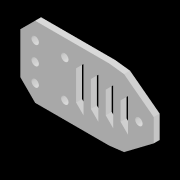
# Autodesk Inventor part: UpperArmMount
Saved by Autodesk Inventor 2020 (Build 240168000, 168)
## iProperties
Created: 2020-03-28
Part Number: UpperArmMount
Material: Generic
Document SubType Name: Modeling
Designer: valer
Density: 1 g/cm^3
Appearance: Default
Author: valer
Autodesk Inventor part; units mm, degrees
ref_plane "YZ Plane" through (0, 0, 0) normal (1, 0, 0) x (0, 1, 0)
ref_plane "XZ Plane" through (0, 0, 0) normal (0, 1, 0) x (-1, 0, 0)
ref_plane "XY Plane" through (0, 0, 0) normal (0, 0, 1) x (1, 0, 0)
sketch "Base" plane through (0, 0, 0) normal (0, 0, 1) x (1, 0, 0)
  line L0 (76.2, -12.7) -> (76.2, -19.05)
  line L1 (0, 0) -> (76.2, 0)
  line L2 (76.2, 0) -> (76.2, -60.96)
  line L3 (76.2, -60.96) -> (0, -60.96)
  line L4 (0, -60.96) -> (0, 0)
  line L5 (76.2, 0) -> (88.9, -1.5594)
  line L6 (88.9, -1.5594) -> (114.3, -20.6996)
  line L7 (114.3, -20.6996) -> (114.3, -30.48)
  line L8 (0, -30.48) -> (114.3, -30.48) construction
  line L9 (76.2, -60.96) -> (88.9, -59.4006)
  line L10 (88.9, -59.4006) -> (114.3, -40.2604)
  line L11 (114.3, -40.2604) -> (114.3, -30.48)
  circle A0 centre (12.7, -46.355) radius 3.175
  circle A1 centre (38.1, -46.355) radius 3.175
  circle A2 centre (38.1, -14.605) radius 3.175
  circle A3 centre (12.7, -14.605) radius 3.175
  line L12 (12.7, -46.355) -> (38.1, -46.355) construction
  line L13 (38.1, -46.355) -> (38.1, -14.605) construction
  line L14 (38.1, -14.605) -> (12.7, -14.605) construction
  line L15 (12.7, -14.605) -> (12.7, -46.355) construction
  circle A4 centre (12.7, -30.48) radius 3.175
  circle A5 centre (101.6, -30.48) radius 3.175
  point P0 (76.2, -30.48)
  dimension "d2" = 76.2
  dimension "d3" = 60.96
  dimension "d4" = 38.1
  dimension "d5" = 12.7
  dimension "d6" = 127
  dimension "d7" = 150
  dimension "d56" = 31.75
  dimension "d57" = 25.4
  dimension "d58" = 12.7
  dimension "d59" = 14.605
  dimension "d60" = 14.605
  dimension "d61" = 6.35
  dimension "d62" = 6.35
  dimension "d63" = 12.7
  constraints: 32 end point, 6 centre point, 4 parallel, 3 coincident, 3 midpoint, 3 point on line, 3 symmetric about line, 2 horizontal, 2 perpendicular, 1 vertical
  measures "d2" distance between parallel lines of L0 L4
  measures "d3" distance of L3.end L1.start
  measures "d4" distance from line of L2 L7.end
  measures "d5" horizontal distance of L1.end L5.end
  measures "d6" angle of L7 L6
  measures "d7" angle of L6 L5
  measures "d56" distance of L14.end L12.start
  measures "d57" distance of L12.start L12.end
  measures "d58" distance between parallel lines of L4 L15
  measures "d59" distance between parallel lines of L3 L12
  measures "d60" distance between parallel lines of L1 L14
  measures "d61" diameter of A4
  measures "d62" diameter of A5
  measures "d63" distance from line of L11 A5.centre
extrude "Extrusion1" add sketch "Base" along normal blind 5.08
chamfer "Chamfer1" distance 12.7 angle 45 2 edges at (0, 0, 2.54) (0, -60.96, 2.54)
sketch "Sketch5" plane through (0, 0, 0) normal (0, 0, -1) x (-1, 0, 0)
  line L0 (0, -12.7) -> (0, -48.26) projected
  line L1 (-47.7822, -17.78) -> (-47.7822, -43.18)
  line L2 (-47.7822, -43.18) -> (-54.1322, -49.53)
  line L3 (-54.1322, -49.53) -> (-54.1322, -11.43)
  line L4 (-54.1322, -11.43) -> (-47.7822, -17.78)
  line L5 (-60.4822, -19.3675) -> (-60.4822, -41.5925)
  line L6 (-60.4822, -19.3675) -> (-66.8322, -13.0175)
  line L7 (-66.8322, -13.0175) -> (-66.8322, -47.9425)
  line L8 (-66.8322, -47.9425) -> (-60.4822, -41.5925)
  line L9 (-54.1322, -11.43) -> (-105.2152, -17.8154) construction
  line L10 (-54.1322, -49.53) -> (-104.6923, -43.21) construction
  line L11 (-79.5322, -14.605) -> (-79.5322, -46.355)
  line L12 (-79.5322, -14.605) -> (-73.1822, -20.955)
  line L13 (-73.1822, -20.955) -> (-73.1822, -40.005)
  line L14 (-73.1822, -40.005) -> (-79.5322, -46.355)
  line L15 (-92.2322, -16.1925) -> (-92.2322, -44.7675)
  line L16 (-92.2322, -44.7675) -> (-85.8822, -38.4175)
  line L17 (-85.8822, -38.4175) -> (-85.8822, -22.5425)
  line L18 (-85.8822, -22.5425) -> (-92.2322, -16.1925)
  line L19 (-47.7822, -30.48) -> (-92.2322, -30.48) construction
  line L20 (0, -30.48) -> (-114.3, -30.48) construction
  line L21 (-114.3, -40.2604) -> (-114.3, -20.6996) projected
  point P0 (-60.4822, -30.48)
  point P1 (-66.8322, -30.48)
  dimension "d34" = 45
  dimension "d35" = 6.35
  dimension "d37" = 38.1
  dimension "d41" = 25.4
  dimension "d42" = 6.35
  dimension "d43" = 6.35
  dimension "d44" = 6.35
  dimension "d45" = 6.35
  dimension "d64" = 82.875
  dimension "d65" = 82.875
  constraints: 40 end point, 6 midpoint, 5 parallel, 5 point on line, 5 vertical, 4 equal length, 1 collinear, 1 horizontal, 1 perpendicular
  measures "d34" angle of L2 L3
  measures "d35" distance between parallel lines of L3 L1
  measures "d37" distance of L2.end L3.end
  measures "d41" distance of L10.end L9.end
  measures "d42" distance between parallel lines of L3 L5
  measures "d43" distance between parallel lines of L7 L5
  measures "d44" distance between parallel lines of L13 L7
  measures "d45" distance between parallel lines of L17 L11
  measures "d64" angle of L9 L3
  measures "d65" angle of L10 L3
extrude "Extrusion2" cut sketch "Sketch5" against normal through all
equation "\"d60\" = d59"
equation "\"d34\" = d31"
equation "\"d35\" = d33"
equation "\"d42\" = d38"
equation "\"d43\" = d40"
equation "\"d44\" = d38"
equation "\"d45\" = d38"
equation "\"d40\" = d33"
equation "\"d31\" = 45deg"
equation "\"d33\" = 6.35"
equation "\"d38\" = 6.35"
body "Solid1"
